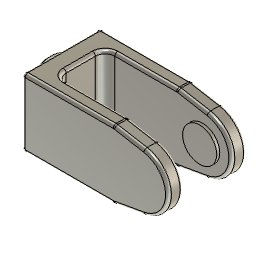
Assembled (Autodesk Fusion 360 archive; units mm, degrees)
design "link4"
part number: 2025-12-13-23-07-16-757
Autodesk Fusion 360 part; units mm, degrees
sketch "Sketch1" plane through (0, 0, 0) normal (0, 1, 0) x (1, 0, 0)
  line L0 (0, 0) -> (0, -70)
  line L1 (0, -70) -> (94.2683, -70)
  line L2 (94.2683, -70) -> (125.2094, -64.5442)
  arc A0 (125.2094, -64.5442) -> (125.2094, -5.4558) centre (120, -35) ccw
  line L3 (125.2094, -5.4558) -> (94.2683, 0)
  line L4 (94.2683, 0) -> (0, 0)
  dimension "d1" = 70
  dimension "d2" = 30
  dimension "d3" = 170
  dimension "d4" = 120
  constraint coincident L0.start L4.end
  constraint vertical L0
  constraint perpendicular L0 L1
  constraint equal L2 L3
  constraint equal L1 L4
  constraint horizontal L4
  constraint tangent L2 A0
  constraint tangent A0 L3
  measures "d1" distance of L0.start L0.end
  measures "d2" radius of A0
  measures "d3" angle of L3 L4
  measures "d4" horizontal distance of L0.start A0.centre
extrude "Extrude1" add sketch "Sketch1" along normal mid plane 80
sketch "Sketch2" plane through (0, 0, 70) normal (0, 0, 1) x (-1, 0, 0)
  line L0 (-94.2683, 40) -> (-94.2683, -40)
  line L1 (-94.2683, -40) -> (0, -40)
  line L2 (0, -40) -> (0, 40)
  line L3 (0, 40) -> (-94.2683, 40)
  line L4 (-20, -25) -> (-190, -25)
  line L5 (-190, -25) -> (-190, 25)
  line L6 (-190, 25) -> (-20, 25)
  line L7 (-20, 25) -> (-20, -25)
  dimension "d7" = 15
  dimension "d8" = 15
  dimension "d9" = 170
  dimension "d10" = 20
  constraint horizontal L4
  constraint vertical L5
  constraint horizontal L6
  constraint vertical L7
  measures "d7" distance of L1 L4.start
  measures "d8" distance of L3 L6
  measures "d9" distance of L5.end L6.end
  measures "d10" distance of L2 L4.start
extrude "Extrude2" cut sketch "Sketch2" against normal through all contours L0 L4 L6 L7 | L0 L4 L5 L6
sketch "Sketch3" plane through (0, 25, 0) normal (0, -1, 0) x (1, 0, 0)
  line L0 (125.2094, 64.5442) -> (94.2683, 70)
  line L1 (94.2683, 70) -> (20, 70)
  line L2 (20, 70) -> (20, 0)
  line L3 (20, 0) -> (94.2683, 0)
  line L4 (94.2683, 0) -> (125.2094, 5.4558)
  arc A0 (125.2094, 5.4558) -> (125.2094, 64.5442) centre (120, 35) ccw
  circle A1 centre (120, 35) radius 17.5
  dimension "d12" = 35
  constraint concentric A0 A1
  measures "d12" diameter of A1
extrude "Extrude3" add sketch "Sketch3" along normal blind 3 contours A1
mirror "Mirror1" about plane through (0, 0, 0) normal (0, 1, 0) of "Extrude3"
sketch "Sketch4" plane through (0, 0, 0) normal (-1, 0, 0) x (0, -1, 0)
  line L0 (40, 70) -> (-40, 70)
  line L1 (-40, 70) -> (-40, 0)
  line L2 (-40, 0) -> (40, 0)
  line L3 (40, 0) -> (40, 70)
  circle A0 centre (0, 35) radius 25
  line L4 (0, 35) -> (-40, 35) construction
  line L5 (0, 35) -> (0, 0) construction
  dimension "d17" = 50
  constraint coincident A0.centre L4.start
  constraint midpoint L1 L4.end
  constraint coincident L5.end origin
  constraint perpendicular L2 L5
  constraint horizontal L4
  measures "d17" diameter of A0
extrude "Extrude4" add sketch "Sketch4" along normal blind 10 contours A0
sketch "Sketch5" plane through (-10, 0, 0) normal (-1, 0, 0) x (0, -1, 0)
  circle A0 centre (0, 35) radius 25
  circle A1 centre (0, 35) radius 22
  dimension "d20" = -3
extrude "Extrude5" add sketch "Sketch5" along normal blind 3 contours A1
fillet "Fillet1" radius 10 6 edges at (20, 25, 35) (20, -25, 35) (94.2683, 32.5, 70) (94.2683, -32.5, 70) (94.2683, -32.5, 0) (94.2683, 32.5, 0)
fillet "Fillet2" radius 3 39 edges at (0, 0, 70) (46.6967, 40, 70) (94.2649, 40, 69.9619) (110.1696, 40, 67.1962) (150, 40, 35) (110.1696, 40, 2.8038) (94.2649, 40, 0.0381) (46.6967, 40, 0) (46.6967, -40, 0) (94.2649, -40, 0.0381) (110.1696, -40, 2.8038) (150, -40, 35) (110.1696, -40, 67.1962) (94.2649, -40, 69.9619) (46.6967, -40, 70) (22.9289, -22.0711, 70) (20, 0, 70) (22.9289, 22.0711, 70) (61.6967, 25, 70) (94.2649, 25, 69.9619) (110.1696, 25, 67.1962) (150, 25, 35) (110.1696, 25, 2.8038) (94.2649, 25, 0.0381) (61.6967, 25, 0) (22.9289, 22.0711, 0) (20, 0, 0) (22.9289, -22.0711, 0) (61.6967, -25, 0) (94.2649, -25, 0.0381) (110.1696, -25, 2.8038) (150, -25, 35) (110.1696, -25, 67.1962) (94.2649, -25, 69.9619) (61.6967, -25, 70) (0, 23.3082, 44.0404) (0, 40, 35) (0, -40, 35) (0, 0, 0)

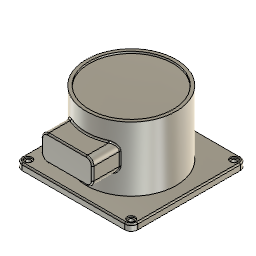
design "Base of robotic arm"
part number: 2025-12-13-21-49-26-084
Autodesk Fusion 360 part; units mm, degrees
sketch "Sketch1" plane through (0, 0, 0) normal (0, 0, 1) x (1, 0, 0)
  line L0 (-90, 90) -> (90, 90)
  line L1 (90, 90) -> (90, -90)
  line L2 (90, -90) -> (-90, -90)
  line L3 (-90, -90) -> (-90, 90)
  line L4 (-90, 90) -> (90, -90) construction
  line L5 (90, 90) -> (-90, -90) construction
  dimension "d1" = 180
  dimension "d2" = 180
  constraint horizontal L0
  constraint perpendicular L0 L1
  constraint parallel L0 L2
  constraint parallel L1 L3
  constraint coincident L4 origin
  constraint coincident L5 origin
  measures "d1" distance of L0.end L1.end
  measures "d2" distance of L0.start L0.end
extrude "Extrude1" add sketch "Sketch1" along normal blind 10
sketch "Sketch2" plane through (0, 0, 10) normal (0, 0, 1) x (-1, 0, 0)
  line L0 (90, 90) -> (-90, 90)
  line L1 (-90, 90) -> (-90, -90)
  line L2 (-90, -90) -> (90, -90)
  line L3 (90, -90) -> (90, 90)
  circle A0 centre (0, 0) radius 70
  dimension "d5" = 140
  constraint coincident A0.centre origin
  measures "d5" diameter of A0
extrude "Extrude2" add sketch "Sketch2" along normal blind 100 contours A0
sketch "Sketch3" plane through (0, 0, 0) normal (0, 1, 0) x (1, 0, 0)
  line L0 (-40, -80) -> (40, -80)
  line L1 (40, -80) -> (40, -40)
  line L2 (40, -40) -> (-40, -40)
  line L3 (-40, -40) -> (-40, -80)
  line L4 (-40, -80) -> (40, -40) construction
  line L5 (40, -80) -> (-40, -40) construction
  point P0 (0, -60)
  dimension "d13" = 40
  dimension "d14" = 80
  dimension "d16" = 60
  constraint horizontal L0
  constraint perpendicular L0 L1
  constraint parallel L0 L2
  constraint parallel L1 L3
  constraint coincident L4 P0
  constraint coincident L5 P0
  measures "d13" distance of L0.start L2.end
  measures "d14" distance of L0.start L0.end
  measures "d16" distance of origin P0
extrude "Extrude3" add sketch "Sketch3" against normal blind 100
sketch "Sketch4" plane through (0, 0, 110) normal (0, 0, 1) x (-1, 0, 0)
  circle A0 centre (0, 0) radius 70
  circle A1 centre (0, 0) radius 65
  dimension "d10" = -5
extrude "Extrude4" cut sketch "Sketch4" against normal blind 10 contours A1
extrude "Extrude5" add 1 faces at (2.3225, -16.9397, 100) along direction (0, 0, 1) blind 7
sketch "Sketch5" plane through (0, 0, 10) normal (0, 0, 1) x (-1, 0, 0)
  circle A0 centre (0, 0) radius 70
  line L0 (90, 90) -> (-90, 90)
  line L1 (-90, 90) -> (-90, -90)
  line L2 (-90, -90) -> (90, -90)
  line L3 (90, -90) -> (90, 90)
  point P0 (80, -80)
  point P1 (-80, -80)
  point P2 (-80, 80)
  point P3 (80, 80)
  point P4 (116.0582, 65.2033)
  dimension "d19" = 10
  dimension "d20" = 10
  dimension "d21" = 10
  dimension "d22" = 10
  dimension "d23" = 10
  dimension "d24" = 10
  dimension "d25" = 10
  dimension "d26" = 10
  constraint horizontal P0 P1
  constraint vertical P1 P2
  constraint horizontal P2 P3
  measures "d19" vertical distance of L0.start P3
  measures "d20" horizontal distance of L0.start P3
  measures "d21" distance of L2 P1
  measures "d22" distance of L1 P1
  measures "d23" vertical distance of L0.start P2
  measures "d24" distance of L1 P2
  measures "d25" distance of L2 P0
  measures "d26" distance of L3 P0
hole "Hole1" at (-80, -80, 10) at (80, -80, 10) at (80, 80, 10) at (-80, 80, 10) direction (0, 0, -1) diameter 7 depth 15 tip angle 118 counterbore diameter 12 counterbore depth 2
fillet "Fillet1" radius 10 8 edges at (-90, -90, 5) (90, -90, 5) (90, 90, 5) (-90, 90, 5) (40, -78.7228, 80) (40, -78.7228, 40) (-40, -78.7228, 80) (-40, -78.7228, 40)
fillet "Fillet2" radius 2 24 edges at (87.0711, -87.0711, 10) (90, 0, 10) (87.0711, 87.0711, 10) (0, 90, 10) (-87.0711, 87.0711, 10) (-90, 0, 10) (-87.0711, -87.0711, 10) (0, -90, 10) (-37.0711, -100, 77.0711) (-40, -100, 60) (-37.0711, -100, 42.9289) (0, -100, 40) (37.0711, -100, 42.9289) (40, -100, 60) (37.0711, -100, 77.0711) (0, -100, 80) (36.9012, -59.4835, 77.2363) (40, -57.4456, 60) (36.9012, -59.4835, 42.7637) (0, -70, 40) (-36.9012, -59.4835, 42.7637) (-40, -57.4456, 60) (-36.9012, -59.4835, 77.2363) (0, -70, 80)

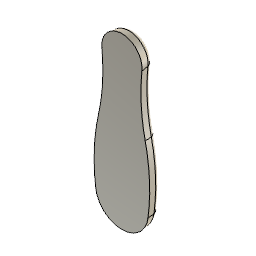
design "link2"
part number: 2025-12-13-22-35-12-355
Autodesk Fusion 360 part; units mm, degrees
sketch "Sketch1" plane through (0, 0, 0) normal (0, 1, 0) x (1, 0, 0)
  arc A0 (35.2531, -100) -> (29.8304, -196.8149) centre (328.1348, -164.9639) ccw
  arc A1 (35.2531, -100) -> (39.6352, 5.3902) centre (-257.6286, -35.0361) ccw
  line L0 (0, -200) -> (0, 0) construction
  arc A2 (-29.8304, -196.8149) -> (-35.2531, -100) centre (-328.1348, -164.9639) ccw
  arc A3 (-39.6352, 5.3902) -> (-35.2531, -100) centre (257.6286, -35.0361) ccw
  arc A4 (-29.8304, -196.8149) -> (29.8304, -196.8149) centre (0, -200) ccw
  arc A5 (39.6352, 5.3902) -> (-39.6352, 5.3902) centre (0, 0) ccw
  dimension "d1" = 80
  dimension "d2" = 60
  dimension "d3" = 200
  dimension "d7" = 100
  dimension "d8" = 300
  constraint coincident L0.end A5.centre
  constraint vertical L0.end L0.start
  constraint tangent A0 A4
  constraint tangent A0 A1
  constraint tangent A1 A5
  constraint coincident L0.start A4.centre
  constraint symmetric A0.end L0 A2.start
  constraint symmetric A0.start L0 A2.end
  constraint symmetric A0 L0 A2
  constraint symmetric A1.end L0 A3.start
  constraint symmetric A1 L0 A3
  constraint equal A0 A1
  measures "d1" diameter of A5
  measures "d2" diameter of A4
  measures "d3" distance of L0.end L0.start
  measures "d7" vertical distance of L0.end A0.start
  measures "d8" radius of A0
extrude "Extrude1" add sketch "Sketch1" against normal blind 20 draft 8
fillet "Fillet1" radius 10 6 edges at (0, 0, 230) (-28.6043, 0, 148.1869) (-42.1125, 0, 47.499) (0, 0, -40) (42.1125, 0, 47.499) (28.6043, 0, 148.1869)

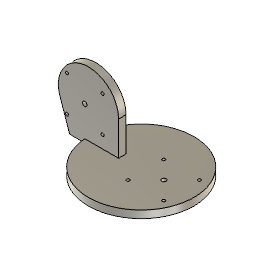
design "link1"
part number: 2025-12-13-21-49-02-726
Autodesk Fusion 360 part; units mm, degrees
sketch "Sketch1" plane through (0, 0, 0) normal (0, 0, 1) x (1, 0, 0)
  circle A0 centre (0, 0) radius 70
  dimension "d1" = 140
  constraint coincident A0.centre origin
  measures "d1" diameter of A0
extrude "Extrude1" add sketch "Sketch1" along normal blind 10
sketch "Sketch2" plane through (0, 0, 0) normal (0, 0, -1) x (1, 0, 0)
  circle A0 centre (0, 0) radius 70
  circle A1 centre (0, 0) radius 65
  dimension "d4" = -5
extrude "Extrude2" add sketch "Sketch2" along normal blind 3 contours A1
sketch "Sketch3" plane through (0, 0, 0) normal (0, 1, 0) x (1, 0, 0)
  line L0 (-25, -55) -> (-25, -5)
  line L1 (-25, -5) -> (-90, -5)
  line L2 (-90, -5) -> (-103.8281, -45.3888)
  arc A0 (-103.8281, -45.3888) -> (-25, -55) centre (-65, -55) ccw
  dimension "d7" = 50
  dimension "d8" = 65
  dimension "d9" = 40
  dimension "d12" = 5
  dimension "d14" = 25
  constraint vertical L0
  constraint perpendicular L0 L1
  constraint tangent L0 A0
  measures "d7" distance of L0.start L0.end
  measures "d8" distance of L0.end L1.end
  measures "d9" radius of A0
  measures "d12" distance of origin L1
  measures "d14" horizontal distance of origin L0.end
extrude "Extrude3" add sketch "Sketch3" along normal mid plane 10
sketch "Sketch4" plane through (0, 0, 10) normal (0, 0, 1) x (-1, 0, 0)
  line L0 (69.8212, -5) -> (25, -5)
  line L1 (25, -5) -> (25, 5)
  line L2 (25, 5) -> (69.8212, 5)
  arc A0 (69.8212, 5) -> (69.8212, -5) centre (0, 0) ccw
  line L3 (-6.378, 23.622) -> (-53.622, 23.622)
  line L4 (-53.622, 23.622) -> (-53.622, -23.622)
  line L5 (-53.622, -23.622) -> (-6.378, -23.622)
  line L6 (-6.378, -23.622) -> (-6.378, 23.622)
  line L7 (-6.378, 23.622) -> (-53.622, -23.622) construction
  line L8 (-53.622, 23.622) -> (-6.378, -23.622) construction
  point P0 (-30, 0)
  dimension "d17" = 47.244
  dimension "d18" = 47.244
  dimension "d20" = 30
  constraint horizontal L3
  constraint perpendicular L3 L4
  constraint parallel L3 L5
  constraint parallel L4 L6
  constraint coincident L7 P0
  constraint coincident L8 P0
  constraint horizontal A0.centre P0
  measures "d17" distance of L3.end L4.end
  measures "d18" distance of L4.end L5.end
  measures "d20" distance of A0.centre P0
hole "Hole1" at (6.378, 23.622, 10) at (53.622, 23.622, 10) at (53.622, -23.622, 10) at (6.378, -23.622, 10) direction (0, 0, -1) diameter 4 depth 15 tip angle 118
hole "Hole2" at (30, 0, 10) direction (0, 0, -1) diameter 6 depth 15 tip angle 118
sketch "Sketch5" plane through (0, -5, 0) normal (0, -1, 0) x (1, 0, 0)
  line L0 (-69.8212, 10) -> (-25, 10)
  line L1 (-25, 10) -> (-25, 55)
  arc A0 (-25, 55) -> (-103.8281, 45.3888) centre (-65, 55) ccw
  line L2 (-103.8281, 45.3888) -> (-90, 5)
  line L3 (-90, 5) -> (-69.8212, 5)
  line L4 (-69.8212, 5) -> (-69.8212, 10)
  line L5 (-93.4432, 73.622) -> (-46.1992, 73.622)
  line L6 (-46.1992, 73.622) -> (-46.1992, 26.378)
  line L7 (-46.1992, 26.378) -> (-93.4432, 26.378)
  line L8 (-93.4432, 26.378) -> (-93.4432, 73.622)
  line L9 (-93.4432, 73.622) -> (-46.1992, 26.378) construction
  line L10 (-46.1992, 73.622) -> (-93.4432, 26.378) construction
  point P0 (-69.8212, 50)
  dimension "d27" = 47.244
  dimension "d28" = 47.244
  dimension "d30" = 45
  constraint horizontal L5
  constraint perpendicular L5 L6
  constraint parallel L5 L7
  constraint parallel L6 L8
  constraint coincident L9 P0
  constraint coincident L10 P0
  constraint vertical L3.end P0
  measures "d27" distance of L5.end L6.end
  measures "d28" distance of L6.end L7.end
  measures "d30" distance of L3 P0
hole "Hole3" at (-93.4432, -5, 73.622) at (-46.1992, -5, 73.622) at (-93.4432, -5, 26.378) at (-46.1992, -5, 26.378) direction (0, 1, 0) diameter 4 depth 15 tip angle 118
hole "Hole4" at (-69.8212, -5, 50) direction (0, 1, 0) diameter 6 depth 15 tip angle 118

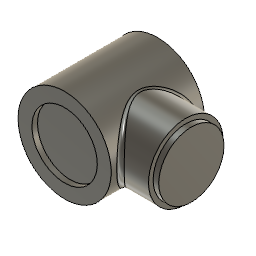
design "link5"
part number: 2025-12-14-18-36-43-908
Autodesk Fusion 360 part; units mm, degrees
sketch "Sketch1" plane through (0, 0, 0) normal (0, 1, 0) x (1, 0, 0)
  circle A0 centre (0, 0) radius 25
  dimension "d1" = 50
  constraint coincident A0.centre origin
  measures "d1" diameter of A0
extrude "Extrude2" add sketch "Sketch1" along normal mid plane 50
sketch "Sketch2" plane through (0, -25, 0) normal (0, -1, 0) x (1, 0, 0)
  circle A0 centre (0, 0) radius 25
  circle A1 centre (0, 0) radius 17.5
  dimension "d6" = 35
  constraint coincident A0.centre A1.centre
  measures "d6" diameter of A1
extrude "Extrude3" cut sketch "Sketch2" against normal blind 3 contours A1
mirror "Mirror1" about plane through (0, 0, 0) normal (0, 1, 0) of "Extrude3"
sketch "Sketch3" plane through (0, 0, 0) normal (1, 0, 0) x (0, 1, 0)
  circle A0 centre (0, 0) radius 20
  dimension "d11" = 40
  constraint coincident A0.centre origin
  measures "d11" diameter of A0
extrude "Extrude4" add sketch "Sketch3" along normal blind 40
sketch "Sketch4" plane through (40, 0, 0) normal (1, 0, 0) x (0, 1, 0)
  circle A0 centre (0, 0) radius 20
  circle A1 centre (0, 0) radius 17.5
  dimension "d14" = 35
  constraint coincident A0.centre A1.centre
  measures "d14" diameter of A1
extrude "Extrude5" add sketch "Sketch4" along normal blind 3 contours A1
fillet "Fillet1" radius 2 1 edges at (15, 0, 20)

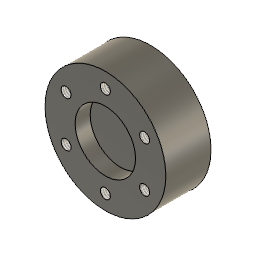
design "link6"
part number: 2025-12-14-18-44-27-514
Autodesk Fusion 360 part; units mm, degrees
sketch "Sketch1" plane through (0, 0, 0) normal (0, 1, 0) x (1, 0, 0)
  circle A0 centre (0, 0) radius 20
  dimension "d1" = 40
  constraint coincident A0.centre origin
  measures "d1" diameter of A0
extrude "Extrude1" add sketch "Sketch1" against normal blind 15
sketch "Sketch2" plane through (0, -15, 0) normal (0, -1, 0) x (1, 0, 0)
  circle A0 centre (0, 0) radius 20
  circle A1 centre (0, 0) radius 10
  dimension "d4" = 20
  constraint coincident A0.centre A1.centre
  measures "d4" diameter of A1
extrude "Extrude2" cut sketch "Sketch2" against normal blind 5 contours A1
sketch "Sketch3" plane through (0, -15, 0) normal (0, -1, 0) x (1, 0, 0)
  circle A0 centre (0, 0) radius 10
  circle A1 centre (0, 0) radius 20
  point P0 (0, 15)
  dimension "d7" = 15
  constraint vertical A0.centre P0
  measures "d7" distance of A0.centre P0
hole "Hole1" at (0, -15, 15) direction (0, 1, 0) diameter 3.332 depth 8 tip angle 118
thread "Thread1" "ISO Metric profile 4.0 M4x0.7 M4x0.7 6H" thread offset 0 thread depth 7.4
pattern_circular "C-Pattern1" count 6 over 360 about axis through (0, 1.75, 0) along (0, 1, 0) of "Hole1"
sketch "Sketch4" plane through (0, 0, 0) normal (0, 1, 0) x (-1, 0, 0)
  circle A0 centre (0, 0) radius 20
  circle A1 centre (0, 0) radius 17.5
  dimension "d15" = 35
  constraint coincident A0.centre A1.centre
  measures "d15" diameter of A1
extrude "Extrude3" cut sketch "Sketch4" against normal blind 3 contours A1

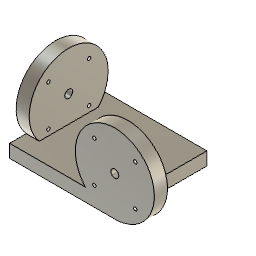
design "link3"
part number: 2025-12-13-22-53-59-055
Autodesk Fusion 360 part; units mm, degrees
sketch "Sketch1" plane through (0, 0, 0) normal (0, 1, 0) x (1, 0, 0)
  circle A0 centre (0, 0) radius 30
  dimension "d1" = 60
  constraint coincident A0.centre origin
  measures "d1" diameter of A0
extrude "Extrude1" add sketch "Sketch1" against normal blind 10
sketch "Sketch2" plane through (0, -10, 0) normal (0, -1, 0) x (1, 0, 0)
  circle A0 centre (0, 0) radius 30
  line L0 (0, -30) -> (-80, -30)
  line L1 (-80, -30) -> (-80, -20)
  line L2 (-80, -20) -> (0, -20)
  line L3 (0, -20) -> (0, -30)
  dimension "d4" = 80
  dimension "d5" = 10
  constraint horizontal L0
  constraint vertical L1
  constraint horizontal L2
  constraint vertical L3
  constraint coincident A0 L0.start
  constraint vertical A0.centre L0.start
  measures "d4" distance of L0.start L0.end
  measures "d5" distance of L0.start L2.end
extrude "Extrude2" add sketch "Sketch2" against normal blind 70 contours A0 L0 L1 L2 | A0 L2 L3 picked at (-1.3972, -26.5686)
sketch "Sketch3" plane through (-80, 0, 0) normal (-1, 0, 0) x (0, -1, 0)
  line L0 (10, -30) -> (10, -20)
  line L1 (10, -20) -> (-60, -20)
  line L2 (-60, -20) -> (-60, -30)
  line L3 (-60, -30) -> (10, -30)
  circle A0 centre (-25, 0) radius 30
  line L4 (-25, 0) -> (-25, -30) construction
  dimension "d8" = 60
  constraint tangent L3 A0
  constraint coincident A0.centre L4.start
  constraint midpoint L3 L4.end
  constraint perpendicular L3 L4
  measures "d8" diameter of A0
extrude "Extrude3" add sketch "Sketch3" against normal blind 10 contours L1 A0 picked at (-17.2718, 11.3343)
sketch "Sketch4" plane through (0, 0, 0) normal (0, 1, 0) x (-1, 0, 0)
  line L0 (0, -30) -> (0, -20)
  line L1 (0, -20) -> (22.3607, -20)
  arc A0 (22.3607, -20) -> (0, -30) centre (0, 0) ccw
  line L2 (-15.5, 15.5) -> (15.5, 15.5)
  line L3 (15.5, 15.5) -> (15.5, -15.5)
  line L4 (15.5, -15.5) -> (-15.5, -15.5)
  line L5 (-15.5, -15.5) -> (-15.5, 15.5)
  line L6 (-15.5, 15.5) -> (15.5, -15.5) construction
  line L7 (15.5, 15.5) -> (-15.5, -15.5) construction
  dimension "d11" = 31
  dimension "d12" = 31
  constraint horizontal L2
  constraint perpendicular L2 L3
  constraint parallel L2 L4
  constraint parallel L3 L5
  constraint coincident L6 A0.centre
  constraint coincident L7 A0.centre
  constraint coincident A0.centre origin
  measures "d11" distance of L3.end L4.end
  measures "d12" distance of L2.end L3.end
hole "Hole1" at (15.5, 0, 15.5) at (-15.5, 0, 15.5) at (15.5, 0, -15.5) at (-15.5, 0, -15.5) direction (0, -1, 0) diameter 2.529 depth 10 tip angle 118
thread "Thread1" "ISO Metric profile 3.0 M3x0.5 M3x0.5 6H" thread offset 0 thread depth 7.4
hole "Hole2" at (0, 0, 0) direction (0, -1, 0) diameter 6 depth 10 tip angle 118
sketch "Sketch5" plane through (-70, 0, 0) normal (1, 0, 0) x (0, 1, 0)
  arc A0 (47.3607, -20) -> (2.6393, -20) centre (25, 0) ccw
  line L0 (2.6393, -20) -> (47.3607, -20)
  line L1 (9.5, 15.5) -> (40.5, 15.5)
  line L2 (40.5, 15.5) -> (40.5, -15.5)
  line L3 (40.5, -15.5) -> (9.5, -15.5)
  line L4 (9.5, -15.5) -> (9.5, 15.5)
  line L5 (9.5, 15.5) -> (40.5, -15.5) construction
  line L6 (40.5, 15.5) -> (9.5, -15.5) construction
  point P0 (25, 0)
  dimension "d21" = 31
  dimension "d22" = 31
  constraint horizontal L1
  constraint perpendicular L1 L2
  constraint parallel L1 L3
  constraint parallel L2 L4
  constraint coincident L5 P0
  constraint coincident L6 P0
  constraint coincident P0 A0.centre
  measures "d21" distance of L2.end L3.end
  measures "d22" distance of L1.end L2.end
hole "Hole3" at (-70, 9.5, 15.5) at (-70, 40.5, 15.5) at (-70, 9.5, -15.5) at (-70, 40.5, -15.5) direction (-1, 0, 0) diameter 2.529 depth 10 tip angle 118
thread "Thread2" "ISO Metric profile 3.0 M3x0.5 M3x0.5 6H" thread offset 0 thread depth 7.4
hole "Hole4" at (-70, 25, 0) direction (-1, 0, 0) diameter 6 depth 10 tip angle 118
